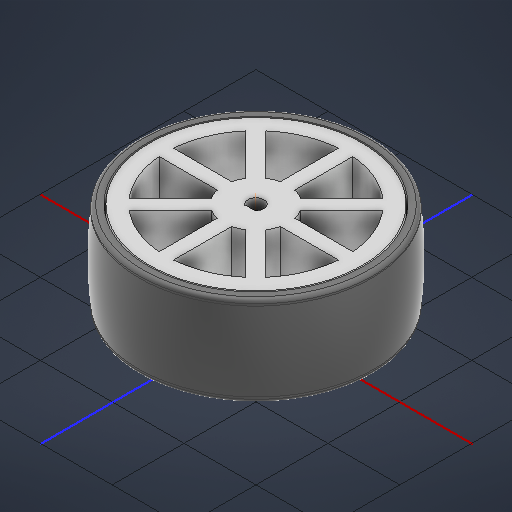
# Autodesk Inventor part: wheel
Saved by Autodesk Inventor 2027 (Build 310192000, 192)
## iProperties
Created: 2026-05-11
Part Number: wheel
Material: Generic
Document SubType Name: Modeling
Designer: maksi
Density: 1 g/cm^3
Appearance: Default
Author: maksi
Autodesk Inventor part; units mm, degrees
ref_plane "YZ Plane" through (0, 0, 0) normal (1, 0, 0) x (0, 1, 0)
ref_plane "XZ Plane" through (0, 0, 0) normal (0, 1, 0) x (-1, 0, 0)
ref_plane "XY Plane" through (0, 0, 0) normal (0, 0, 1) x (1, 0, 0)
sketch "Sketch1" plane through (0, 0, 0) normal (0, 1, 0) x (-1, 0, 0)
  circle A0 centre (-0.022703, 0.034055) radius 32.5
  arc A1 (-1.345579, 1.534055) -> (1.300172, 1.534055) centre (-0.022703, 0.034055) ccw
  line L0 (1.300172, 1.534055) -> (-1.345579, 1.534055)
  arc A2 (-1.419127, 1.734055) -> (1.373721, 1.734055) centre (-0.022703, 0.034055) ccw
  line L1 (-1.419127, 1.734055) -> (1.373721, 1.734055)
  circle A3 centre (-0.022703, 0.034055) radius 29.5
  circle A4 centre (-0.022703, 0.034055) radius 29.875
  circle A5 centre (1.373721, 1.734055) radius 0.1
  circle A6 centre (-1.419127, 1.734055) radius 0.1
  point P0 (0, 0)
  point P1 (-1.494938, 1.668842)
  point P2 (-1.319127, 1.734055)
  point P3 (1.273721, 1.734055)
  point P4 (1.449531, 1.668842)
  dimension "d0" = 65
  dimension "d1" = 0.2
  dimension "d2" = 59
  dimension "d3" = 59.75
  dimension "d9" = 0.2
  dimension "d10" = 0.2
  constraints: 7 centre point, 4 coincident, 4 end point, 4 point on circle, 1 other
  measures "d0" diameter of A0
  measures "d1" radial gap between concentric circles of A1 A2
  measures "d2" diameter of A3
  measures "d3" diameter of A4
  measures "d9" diameter of A5
  measures "d10" diameter of A6
extrude "Extrusion1" add sketch "Sketch1" along normal blind 25 contours A3
extrude "Extrusion2" add sketch "Sketch1" along normal blind 25 contours A0
fillet "Fillet1" radius 1 2 edges at (32.5227, 25, 0.0341) (32.5227, 0, 0.0341)
sketch "Sketch2" plane through (0.022703, 25, 0.034055) normal (0, 1, 0) x (1, 0, 0)
  circle A0 centre (-0.022703, 0.034055) radius 9
  circle A1 centre (-0.022703, 0.034055) radius 25
  line L0 (-18.03925, 20.819516) -> (20.851623, -18.071357)
  line L1 (20.851623, -18.071357) -> (18.023196, -20.899784)
  line L2 (18.023196, -20.899784) -> (-20.867677, 17.991088)
  line L3 (-20.867677, 17.991088) -> (-18.03925, 20.819516)
  line L4 (27.477297, -1.965945) -> (-27.522703, 2.034055) construction
  line L5 (-27.522703, -1.965945) -> (27.477297, 2.034055) construction
  line L6 (1.977297, -27.465945) -> (-2.022703, -27.465945)
  line L7 (-2.022703, -27.465945) -> (-2.022703, 27.534055)
  line L8 (-2.022703, 27.534055) -> (1.977297, 27.534055)
  line L9 (1.977297, 27.534055) -> (1.977297, -27.465945)
  line L10 (1.977297, -27.465945) -> (-2.022703, 27.534055) construction
  line L11 (-2.022703, -27.465945) -> (1.977297, 27.534055) construction
  line L12 (27.477297, -1.965945) -> (-27.522703, -1.965945)
  line L13 (-27.522703, -1.965945) -> (-27.522703, 2.034055)
  line L14 (-27.522703, 2.034055) -> (27.477297, 2.034055)
  line L15 (27.477297, 2.034055) -> (27.477297, -1.965945)
  line L16 (27.477297, -1.965945) -> (-27.522703, 2.034055) construction
  line L17 (-27.522703, -1.965945) -> (27.477297, 2.034055) construction
  line L18 (-20.819516, -18.03925) -> (18.071357, 20.851623)
  line L19 (18.071357, 20.851623) -> (20.899784, 18.023196)
  line L20 (20.899784, 18.023196) -> (-17.991088, -20.867677)
  line L21 (-17.991088, -20.867677) -> (-20.819516, -18.03925)
  point P0 (1.977297, -8.740909)
  point P1 (1.977297, -24.885816)
  point P2 (16.151923, -19.028512)
  point P3 (4.731306, -7.607894)
  point P4 (24.897168, -1.965945)
  point P5 (8.752261, -1.965945)
  point P6 (7.573298, -4.793032)
  point P7 (18.985127, -16.204861)
  point P8 (19.060691, 16.184103)
  point P9 (7.636616, 4.760028)
  point P10 (8.752261, 2.034055)
  point P11 (24.897168, 2.034055)
  point P12 (4.832104, 7.612369)
  point P13 (16.240685, 19.020951)
  point P14 (1.977297, 24.953927)
  point P15 (1.977297, 8.80902)
  point P16 (-2.022703, 8.80902)
  point P17 (-2.022703, 24.953927)
  point P18 (-16.26162, 19.041885)
  point P19 (-4.84979, 7.630056)
  point P20 (-24.942575, 2.034055)
  point P21 (-8.797668, 2.034055)
  point P22 (-7.664653, 4.788065)
  point P23 (-19.08527, 16.208682)
  point P24 (-19.009599, -16.229333)
  point P25 (-7.601018, -4.820752)
  point P26 (-8.797668, -1.965945)
  point P27 (-24.942575, -1.965945)
  point P28 (-4.748676, -7.625265)
  point P29 (-16.172751, -19.04934)
  point P30 (-2.022703, -24.885816)
  point P31 (-2.022703, -8.740909)
  dimension "d11" = 18
  dimension "d12" = 50
  dimension "d13" = 55
  dimension "d14" = 4
  dimension "d15" = 4
  dimension "d16" = 55
  constraints: 44 end point, 8 parallel, 6 midpoint, 4 perpendicular, 2 centre point, 2 coincident, 2 horizontal
  measures "d11" diameter of A0
  measures "d12" diameter of A1
  measures "d13" distance of L1.end L2.end
  measures "d14" distance of L0.end L1.end
  measures "d15" distance of L7.end L8.end
  measures "d16" distance of L6.end L7.end
extrude "Extrusion3" cut sketch "Sketch2" against normal blind 25 contours A0 L20 A1 L14 | L12 A1 L0 A0 | A0 L9 A1 L18 | L2 A1 L9 A0 | A0 L0 A1 L7 | L7 A1 L20 A0 | A0 L14 A1 L2 | L18 A1 L12 A0
ref_plane "Work Plane1" through (-24.919872, 25, 0) normal (0, 0, 1) x (1, 0, 0)
sketch "Sketch3" plane through (-24.919872, 25, 0) normal (0, 0, 1) x (1, 0, 0)
  line L0 (-7.557425, -24) -> (-7.557425, -1)
  line L1 (57.442575, -24) -> (57.442575, -1)
  line L2 (57.442575, -1) -> (-7.557425, -1)
  line L3 (-7.557425, -1) -> (-7.557425, -24)
  line L4 (-7.557425, -24) -> (57.442575, -24)
  line L5 (57.442575, -24) -> (57.442575, -1)
  arc A0 (-7.557425, -1) -> (-7.557425, -24) centre (92.849951, -12.5) ccw
  line L6 (-7.557425, -1) -> (57.442575, -24) construction
  line L7 (-7.557425, -24) -> (57.442575, -1) construction
  line L8 (26.414809, -25) -> (26.414809, 0) construction
  line L9 (26.414809, -13.020944) -> (26.414809, -1) construction
  line L10 (26.414809, -13.020944) -> (26.414809, -24) construction
  line L11 (24.919872, -30) -> (24.919872, 5)
  point P0 (24.919872, -25)
  constraints: 16 end point, 7 point on line, 2 parallel, 2 perpendicular, 2 point on circle, 1 centre point
revolve "Revolution1" add sketch "Sketch3" angle 360 about axis through (0, -10, 0) along (0, 1, 0) contours A0 L0
extrude "Extrusion4" add sketch "Sketch1" along normal blind 7.5 contours L0 A1 | L1 A6 A2 | A2 A6 L1 | A6 L1 A5 A2 | A5 L1 A2 | A2 L1 A5
body "Solid1"
